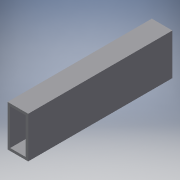
# Autodesk Inventor part: Motor Mount 2
Saved by Autodesk Inventor 2018 (Build 220112000, 112)
## iProperties
Created: 2018-01-29
Part Number: Motor Mount 2
Material: Generic
Document SubType Name: Modeling
Designer: Apple
Density: 1 g/cm^3
Appearance: Default
Author: Apple
Autodesk Inventor part; units mm, degrees
ref_plane "YZ Plane" through (0, 0, 0) normal (1, 0, 0) x (0, 1, 0)
ref_plane "XZ Plane" through (0, 0, 0) normal (0, 1, 0) x (-1, 0, 0)
ref_plane "XY Plane" through (0, 0, 0) normal (0, 0, 1) x (1, 0, 0)
sketch "Sketch1" plane through (0, 0, 0) normal (0, 0, 1) x (1, 0, 0)
  line L0 (-61.9417, 182.4966) -> (-36.5417, 182.4966)
  line L1 (-36.5417, 182.4966) -> (-36.5417, 131.6966)
  line L2 (-36.5417, 131.6966) -> (-61.9417, 131.6966)
  line L3 (-61.9417, 131.6966) -> (-61.9417, 182.4966)
  line L4 (-58.7667, 179.3216) -> (-39.7167, 179.3216)
  line L5 (-39.7167, 179.3216) -> (-39.7167, 134.8716)
  line L6 (-39.7167, 134.8716) -> (-58.7667, 134.8716)
  line L7 (-58.7667, 134.8716) -> (-58.7667, 179.3216)
  point P0 (0, 0)
  dimension "d0" = 25.4
  dimension "d1" = 50.8
  dimension "d2" = 3.175
  constraints: 16 end point, 4 parallel, 2 perpendicular, 1 horizontal, 3 other
  measures "d0" distance of L0.start L0.end
  measures "d1" distance of L2.end L0.start
  measures "d2" distance between parallel lines of L3 L7
extrude "Extrusion1" add sketch "Sketch1" against normal blind 177.8
body "Solid1"
